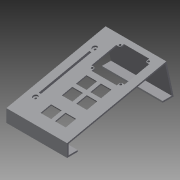
# Autodesk Inventor part: Main_Corpse
Saved by Autodesk Inventor 2015 (Build 190159000, 159)
## iProperties
Created: 2022-04-16
Part Number: Main_Corpse
Material: Generic
Document SubType Name: Modeling
Designer: Jan
Density: 1 g/cm^3
Appearance: Default
Author: Jan
Autodesk Inventor part; units mm, degrees
ref_plane "YZ Plane" through (0, 0, 0) normal (1, 0, 0) x (0, 1, 0)
ref_plane "XZ Plane" through (0, 0, 0) normal (0, 1, 0) x (-1, 0, 0)
ref_plane "XY Plane" through (0, 0, 0) normal (0, 0, 1) x (1, 0, 0)
sketch "Sketch2" plane through (0, 0, 0) normal (1, 0, 0) x (0, 1, 0)
  line L0 (14, 0) -> (0, 0)
  line L1 (0, 0) -> (0, 16.8)
  line L2 (0, 16.8) -> (130.6501, 44.8)
  line L3 (130.6501, 44.8) -> (140.2513, 0)
  line L4 (140.2513, 0) -> (125.7773, 0)
  line L5 (125.7773, 0) -> (125.7773, 2)
  line L6 (125.7773, 2) -> (137.7773, 2)
  line L7 (137.7773, 2) -> (129.1136, 42.4253)
  line L8 (129.1136, 42.4253) -> (2, 15.1832)
  line L9 (2, 15.1832) -> (2, 2)
  line L10 (2, 2) -> (14, 2)
  line L11 (14, 2) -> (14, 0)
  dimension "d0" = 2
  dimension "d1" = 2
  dimension "d2" = 2
  dimension "d3" = 2
  dimension "d4" = 12
  dimension "d5" = 12
  dimension "d6" = 130
  dimension "d7" = 16.8
  dimension "d8" = 44.8
  constraints: 24 end point, 6 perpendicular, 2 parallel, 2 point on line, 1 coincident, 1 collinear, 1 horizontal
  measures "d0" distance between parallel lines of L8 L2
  measures "d1" distance between parallel lines of L7 L3
  measures "d2" distance between parallel lines of L4 L6
  measures "d3" distance between parallel lines of L1 L9
  measures "d4" distance from line of L5 L6.end
  measures "d5" distance between parallel lines of L9 L11
  measures "d6" distance of L7.end L8.end
  measures "d7" distance of L0.end L1.end
  measures "d8" distance from line of L2.end L4
extrude "Extrusion1" add sketch "Sketch2" along normal blind 80
sketch "Sketch3" plane through (0, 0, 16.8) normal (0, -0.2095545, 0.977797) x (1, 0, 0)
  circle A0 centre (12, 106.8084) radius 1.3
  circle A1 centre (12, 26.8084) radius 1.3
  line L0 (0, 133.6168) -> (80, 133.6168) projected
  line L1 (0, 0) -> (80, 0) projected
  line L2 (12, 133.6168) -> (12, 106.8084) construction
  line L3 (12, 0) -> (12, 26.8084) construction
  line L4 (45.05, 75.9904) -> (31.05, 75.9904)
  line L5 (31.05, 75.9904) -> (31.05, 61.9904)
  line L6 (31.05, 61.9904) -> (45.05, 61.9904)
  line L7 (45.05, 61.9904) -> (45.05, 75.9904)
  line L8 (64.1, 75.9904) -> (50.1, 75.9904)
  line L9 (50.1, 75.9904) -> (50.1, 61.9904)
  line L10 (50.1, 61.9904) -> (64.1, 61.9904)
  line L11 (64.1, 61.9904) -> (64.1, 75.9904)
  line L12 (45.05, 56.9404) -> (31.05, 56.9404)
  line L13 (31.05, 56.9404) -> (31.05, 42.9404)
  line L14 (31.05, 42.9404) -> (45.05, 42.9404)
  line L15 (45.05, 42.9404) -> (45.05, 56.9404)
  line L16 (64.1, 56.9404) -> (50.1, 56.9404)
  line L17 (50.1, 56.9404) -> (50.1, 42.9404)
  line L18 (50.1, 42.9404) -> (64.1, 42.9404)
  line L19 (64.1, 42.9404) -> (64.1, 56.9404)
  line L20 (3, 119.3084) -> (21, 119.3084)
  line L21 (21, 119.3084) -> (21, 12.8084)
  line L22 (21, 12.8084) -> (3, 12.8084)
  line L23 (3, 12.8084) -> (3, 119.3084)
  line L24 (3, 66.8084) -> (21, 66.8084) construction
  line L25 (10.6, 100.8084) -> (13.4, 100.8084)
  line L26 (13.4, 100.8084) -> (13.4, 32.8084)
  line L27 (13.4, 32.8084) -> (10.6, 32.8084)
  line L28 (10.6, 32.8084) -> (10.6, 100.8084)
  line L29 (0, 0) -> (0, 133.6168) construction
  line L30 (31.05, 28.3654) -> (45.05, 28.3654)
  line L31 (45.05, 28.3654) -> (45.05, 14.3654)
  line L32 (45.05, 14.3654) -> (31.05, 14.3654)
  line L33 (31.05, 14.3654) -> (31.05, 28.3654)
  line L34 (50.1, 28.3654) -> (64.1, 28.3654)
  line L35 (64.1, 28.3654) -> (64.1, 14.3654)
  line L36 (64.1, 14.3654) -> (50.1, 14.3654)
  line L37 (50.1, 14.3654) -> (50.1, 28.3654)
  line L38 (12, 26.8084) -> (21, 26.8084) construction
  line L39 (24.575, 81.6168) -> (70.575, 81.6168)
  line L40 (70.575, 81.6168) -> (70.575, 128.6168)
  line L41 (70.575, 128.6168) -> (24.575, 128.6168)
  line L42 (24.575, 128.6168) -> (24.575, 81.6168)
  line L43 (47.575, 128.6168) -> (47.575, 37.1123) construction
  line L44 (0, 131.6168) -> (80, 131.6168) projected
  line L45 (0, 131.6168) -> (80, 131.6168) projected
  line L46 (25.775, 126.666) -> (69.375, 126.666)
  line L47 (69.375, 126.666) -> (69.375, 83.066)
  line L48 (25.775, 83.066) -> (25.775, 126.666)
  circle A2 centre (28.825, 123.616) radius 1.4
  circle A3 centre (66.325, 123.616) radius 1.4
  circle A4 centre (66.325, 86.116) radius 1.4
  circle A5 centre (28.825, 86.116) radius 1.4
  line L49 (25.775, 121.466) -> (28.825, 121.466)
  line L50 (30.975, 126.666) -> (30.975, 123.616)
  line L51 (64.175, 126.666) -> (64.175, 123.616)
  line L52 (69.375, 121.466) -> (66.325, 121.466)
  line L53 (25.775, 83.066) -> (69.375, 83.066)
  line L54 (30.975, 83.066) -> (30.975, 86.116)
  line L55 (25.775, 88.266) -> (28.825, 88.266)
  line L56 (69.375, 88.266) -> (66.325, 88.266)
  line L57 (64.175, 83.066) -> (64.175, 86.116)
  arc A6 (28.825, 121.466) -> (30.975, 123.616) centre (28.825, 123.616) ccw
  arc A7 (64.175, 123.616) -> (66.325, 121.466) centre (66.325, 123.616) ccw
  arc A8 (66.325, 88.266) -> (64.175, 86.116) centre (66.325, 86.116) ccw
  arc A9 (30.975, 86.116) -> (28.825, 88.266) centre (28.825, 86.116) ccw
  point P0 (0, -3.5205)
  dimension "d12" = 2.6
  dimension "d14" = 80
  dimension "d15" = 14
  dimension "d23" = 19.05
  dimension "d26" = 19.05
  dimension "d29" = 54
  dimension "d30" = 52.5
  dimension "d31" = 18
  dimension "d33" = 68
  dimension "d34" = 2.8
  dimension "d35" = 12
  dimension "d37" = 28.575
  dimension "d39" = 19.05
  dimension "d42" = 47
  dimension "d43" = 46
  dimension "d56" = 3
  dimension "d57" = 43.6
  dimension "d58" = 37.5
  dimension "d59" = 37.5
  dimension "d60" = 2.8
  dimension "d61" = 5.2
  constraints: 106 end point, 14 point on line, 13 parallel, 12 horizontal, 11 collinear, 11 perpendicular, 10 centre point, 8 point on circle, 8 tangent, 8 vertical, 5 equal length, 4 concentric, 4 equal radius, 3 vertical alignment, 2 horizontal alignment, 2 symmetric about line, 1 midpoint, 28 other
  measures "d12" diameter of A0
  measures "d14" distance of L2.end L3.end
  measures "d15" distance between parallel lines of L5 L7
  measures "d23" distance of L4.start L8.start
  measures "d26" distance of L4.start L12.start
  measures "d29" distance between parallel lines of L22 L24
  measures "d30" distance between parallel lines of L20 L24
  measures "d31" distance between parallel lines of L21 L23
  measures "d33" distance between parallel lines of L27 L25
  measures "d34" distance between parallel lines of L26 L28
  measures "d35" distance between parallel lines of L29 L2
  measures "d37" distance between parallel lines of L14 L32
  measures "d39" distance between parallel lines of L33 L3
  measures "d42" distance between parallel lines of L39 L41
  measures "d43" distance between parallel lines of L40 L42
  measures "d56" distance between parallel lines of L44 L41
  measures "d57" distance between parallel lines of L47 L48
  measures "d58" distance of A4.centre A3.centre
  measures "d59" distance of A3.centre A2.centre
  measures "d60" diameter of A2
  measures "d61" distance between parallel lines of L46 L49
extrude "Extrusion2" cut sketch "Sketch3" against normal up to next contours A0 | A1 | L7 L6 L5 L4 | L11 L10 L9 L8 | L15 L14 L13 L12 | L19 L18 L17 L16 | L25 L26 L27 L28 | L30 L31 L32 L33 | L34 L35 L36 L37 | L46 L51 A7 L52 L47 L56 A8 L57 L53 L54 A9 L55 L48 L49 A6 L50 | A2 | A3 | A4 | A5
sketch "Sketch4" plane through (80, 129.1136, 42.4253) normal (0, 0.2095545, -0.977797) x (-1, 0, 0)
  line L0 (12.9, -52.6264) -> (51.95, -52.6264)
  line L1 (51.95, -52.6264) -> (51.95, -120.2514)
  line L2 (51.95, -120.2514) -> (12.9, -120.2514)
  line L3 (12.9, -120.2514) -> (12.9, -52.6264)
  line L4 (15.9, -55.6264) -> (29.9, -55.6264) projected
  line L5 (15.9, -69.6264) -> (15.9, -55.6264) projected
  line L6 (48.95, -103.2514) -> (48.95, -117.2514) projected
  line L7 (48.95, -117.2514) -> (34.95, -117.2514) projected
  point P0 (80, -135.1373)
  dimension "d44" = 3
  dimension "d45" = 3
  dimension "d46" = 3
  dimension "d47" = 3
  constraints: 8 end point, 2 parallel, 1 horizontal, 1 perpendicular
  measures "d44" distance between parallel lines of L3 L5
  measures "d45" distance between parallel lines of L0 L4
  measures "d46" distance between parallel lines of L1 L6
  measures "d47" distance between parallel lines of L7 L2
extrude "Extrusion3" cut sketch "Sketch4" against normal blind 0.4
extrude "Extrusion4" add sketch "Sketch3" against normal blind 3.6 contours L20 L21 L22 L23
sketch "Sketch6" plane through (0, 0, 16.8) normal (0, -0.2095545, 0.977797) x (1, 0, 0)
  circle A0 centre (12, 26.8084) radius 1.3 projected
  circle A1 centre (12, 106.8084) radius 1.3 projected
  circle A2 centre (12, 26.8084) radius 3.2
  circle A3 centre (12, 106.8084) radius 3.2
  point P0 (0, -3.5205)
  dimension "d52" = 6.4
  constraints: 2 centre point, 2 coincident, 1 equal radius
  measures "d52" diameter of A2
extrude "Extrusion5" cut sketch "Sketch6" against normal blind 2
body "Solid1"
